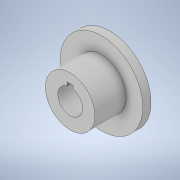
# Autodesk Inventor part: SprocketAdapter
Saved by Autodesk Inventor 2021 (Build 250183000, 183)
## iProperties
Created: 2020-09-20
Part Number: SprocketAdapter
Material: Generic
Document SubType Name: Modeling
Designer: PhotonUser
Density: 1 g/cm^3
Appearance: Default
Author: PhotonUser
Autodesk Inventor part; units mm, degrees
ref_plane "YZ Plane" through (0, 0, 0) normal (1, 0, 0) x (0, 1, 0)
ref_plane "XZ Plane" through (0, 0, 0) normal (0, 1, 0) x (-1, 0, 0)
ref_plane "XY Plane" through (0, 0, 0) normal (0, 0, 1) x (1, 0, 0)
sketch "Sketch1" plane through (0, 0, 0) normal (1, 0, 0) x (0, 1, 0)
  line L0 (0, 0) -> (19.05, 0)
  line L1 (19.05, 0) -> (19.05, -24.13)
  line L2 (19.05, -24.13) -> (31.75, -24.13)
  line L3 (31.75, -24.13) -> (31.75, -30.48)
  line L4 (31.75, -30.48) -> (0, -30.48)
  line L5 (0, -30.48) -> (0, 0)
  dimension "d0" = 19.05
  dimension "d1" = 24.13
  dimension "d2" = 12.7
  dimension "d3" = 6.35
  constraints: 12 end point, 3 perpendicular, 2 horizontal, 1 vertical
  measures "d0" distance of L0.start L0.end
  measures "d1" distance of L0.end L1.end
  measures "d2" distance of L1.end L2.end
  measures "d3" distance of L2.end L3.end
revolve "Revolution1" add sketch "Sketch1" angle 360 about axis through (0, 0, -30.48) along (0, 0, 1)
sketch "Sketch2" plane through (0, 0, 0) normal (0, 0, 1) x (1, 0, 0)
  circle A0 centre (0, 0) radius 9.525
  line L0 (-2.3876, 9.2209) -> (-2.3876, 11.7609)
  line L1 (-2.3876, 11.7609) -> (2.3876, 11.7609)
  line L2 (2.3876, 11.7609) -> (2.3876, 9.2209)
  line L3 (0, 0) -> (0, 17.9613)
  point P0 (0, 11.7609)
  dimension "d5" = 19.05
  dimension "d6" = 4.7752
  dimension "d7" = 2.54
  constraints: 8 end point, 2 perpendicular, 2 point on circle, 2 vertical, 1 centre point, 1 coincident, 1 midpoint, 1 point on line
  measures "d5" diameter of A0
  measures "d6" distance of L0.end L1.end
  measures "d7" distance from line of L1 L0.start
extrude "Extrusion1" cut sketch "Sketch2" against normal through all
body "Solid1"
